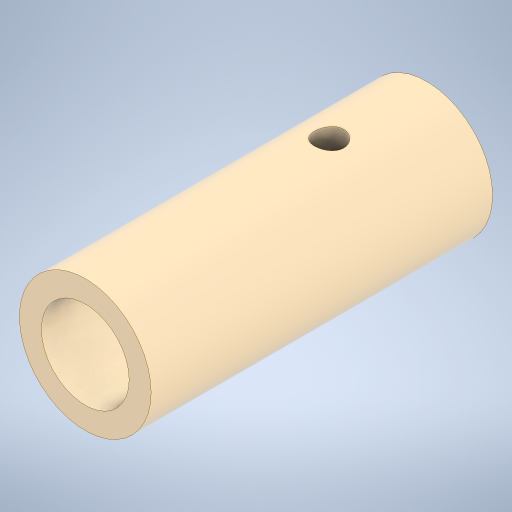
# Autodesk Inventor part: HUDSON-1-74
Saved by Autodesk Inventor 2024.2 (Build 282272000, 272)
## iProperties
Created: 2024-09-29
Part Number: HUDSON-1-74
Material: Generic
Document SubType Name: Modeling
Designer: melim
Density: 1 g/cm^3
Appearance: Smooth - Off-White
Author: melim
Autodesk Inventor part; units mm, degrees
note: some values were not read from the file. Chosen so that the rebuilt part matches the saved one: direction of "Hole2".
ref_plane "YZ Plane" through (0, 0, 0) normal (1, 0, 0) x (0, 1, 0)
ref_plane "XY Plane" through (0, 0, 0) normal (0, 0, 1) x (1, 0, 0)
sketch "Sketch1" plane through (0, 0, 0) normal (0, 0, 1) x (1, 0, 0)
  circle A0 centre (0, 0) radius 6.75
  dimension "d0" = 13.5
  constraints: 1 centre point, 1 coincident
  measures "d0" diameter of A0
extrude "Extrusion1" add sketch "Sketch1" along normal blind 35
sketch "Sketch2" plane through (0, 0, 35) normal (0, 0, 1) x (1, 0, 0)
  point P0 (0, 0)
hole "Hole1" at (0, 0, 35) direction (0, 0, -1) diameter 9 end through all
ref_plane "Work Plane1" through (0, 6.75, 0) normal (0, 1, 0) x (-1, 0, 0)
sketch "Sketch3" plane through (0, 6.75, 0) normal (0, 1, 0) x (-1, 0, 0)
  line L0 (6.75, 0) -> (-6.75, 0) projected
  point P0 (0, 0)
  point P1 (0, 10)
  dimension "d10" = 10
  dimension "d11" = 6.75
  measures "d10" distance from line of point (0, 10) L0
  measures "d11" horizontal distance of L0.start point (0, 10)
hole "Hole2" at (0, 6.75, 10) direction (0, -1, 0) diameter 3 end up to surface
body "Solid1"
